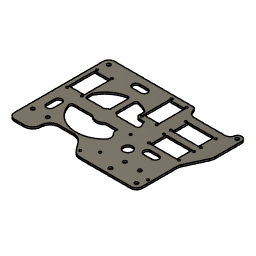
3_Superior (Autodesk Fusion 360 design; units mm, degrees)
Autodesk Fusion 360 part; units mm, degrees
sketch "Sketch1" plane through (0, 0, 0) normal (0, 1, 0) x (1, 0, 0)
  line L0 (40.357, -84) -> (129, -84)
  circle A0 centre (134, -59) radius 2
  arc A1 (35.9352, -34.7659) -> (35.1217, -20.107) centre (28.7481, -27.8127) ccw
  circle A2 centre (31, -74) radius 2
  arc A3 (129, -84) -> (139, -74) centre (129, -74) ccw
  circle A4 centre (51, -59) radius 2
  arc A5 (28.5369, -78.2349) -> (40.357, -84) centre (40.357, -69) ccw
  line L1 (11.1803, -10) -> (32.2785, -10)
  circle A6 centre (129, -74) radius 3
  arc A7 (32.2785, -10) -> (35.1217, -20.107) centre (41, -13) ccw
  circle A8 centre (-73, -52) radius 3
  arc A9 (-56, -84) -> (-41, -69) centre (-56, -69) ccw
  circle A10 centre (-73, 80) radius 3
  line L2 (-83, 80) -> (-83, -74)
  line L3 (-5, 45.111) -> (-5, 14.1421)
  arc A11 (9.7826, 49.0337) -> (5, 45.111) centre (9, 45.111) ccw
  arc A12 (-5, 14.1421) -> (-11.1803, 10) centre (0, 0) ccw
  arc A13 (-44.3962, 10.042) -> (-43.8178, 10) centre (-43.8178, 14) ccw
  arc A14 (-83, -74) -> (-73, -84) centre (-73, -74) ccw
  arc A15 (15.608, -61.6868) -> (-0.1522, -54) centre (-0.1522, -74) ccw
  arc A16 (-11.1803, -10) -> (11.1803, -10) centre (0, 0) ccw
  line L4 (63.3347, 90) -> (-73, 90)
  line L5 (-11.1803, 10) -> (-41.3962, 10)
  arc A17 (-5, 45.111) -> (-9.7826, 49.0337) centre (-9, 45.111) ccw
  line L6 (-73, -84) -> (-56, -84)
  line L7 (-68.3571, -32.6664) -> (-68.3571, -18.3202)
  circle A18 centre (-47, -52) radius 3
  arc A19 (-68.3571, -32.6664) -> (-56.1475, -32.6664) centre (-62.2523, -32.6664) ccw
  line L8 (-43.8178, -10) -> (-11.1803, -10)
  line L9 (43.8178, 10) -> (11.1803, 10)
  arc A20 (43.8178, 10) -> (47.628, 15.2174) centre (43.8178, 14) ccw
  circle A21 centre (51, -6) radius 2
  line L10 (15.608, -61.6868) -> (28.5369, -78.2349)
  circle A22 centre (84, -74) radius 3
  arc A23 (-26, -54) -> (-41, -69) centre (-26, -69) ccw
  line L11 (-56.1475, -18.3202) -> (-56.1475, -32.6664)
  arc A24 (-9.7826, 49.0337) -> (-44.3962, 22.9996) centre (0, 0) ccw
  arc A25 (-56.1475, -18.3202) -> (-68.3571, -18.3202) centre (-62.2523, -18.3202) ccw
  arc A26 (11.1803, 10) -> (5, 14.1421) centre (0, 0) ccw
  line L12 (5, 14.1421) -> (5, 45.111)
  arc A27 (-43.8178, -10) -> (-47.628, -15.2174) centre (-43.8178, -14) ccw
  line L13 (-26, -54) -> (-0.1522, -54)
  arc A28 (-47.628, -15.2174) -> (35.9352, -34.7659) centre (0, 0) ccw
  arc A29 (-73, 90) -> (-83, 80) centre (-73, 80) ccw
  circle A30 centre (150, 80) radius 3
  line L14 (67.95, 86.9234) -> (70.7446, 80.2178)
  arc A31 (70.7446, 80.2178) -> (80.7256, 74.43) centre (80.7256, 85.93) ccw
  line L15 (80.7256, 74.43) -> (134, 74.43)
  arc A32 (134, 74.43) -> (143.5, 83.93) centre (134, 83.93) ccw
  line L16 (157.5957, 80) -> (157.5957, 34.3748)
  line L17 (155.7692, 26.0247) -> (140.8265, -6.4974)
  line L18 (139, -74) -> (139, -14.8474)
  arc A33 (67.95, 86.9234) -> (63.3347, 90) centre (63.3347, 85) ccw
  arc A34 (155.7692, 26.0247) -> (157.5957, 34.3748) centre (137.5957, 34.3748) ccw
  arc A35 (140.8265, -6.4974) -> (139, -14.8474) centre (159, -14.8474) ccw
  arc A36 (157.5957, 80) -> (143.5, 83.93) centre (150, 80) ccw
  arc A37 (78.8091, 65.3966) -> (73.3091, 59.8966) centre (78.8091, 59.8966) ccw construction
  line L19 (73.3091, 59.8966) -> (73.3091, 36.8966) construction
  arc A38 (73.3091, 36.8966) -> (78.8091, 31.3966) centre (78.8091, 36.8966) ccw construction
  line L20 (78.8091, 31.3966) -> (131.8091, 31.3966) construction
  arc A39 (131.8091, 31.3966) -> (137.3091, 36.8966) centre (131.8091, 36.8966) ccw construction
  line L21 (137.3091, 36.8966) -> (137.3091, 59.8966) construction
  arc A40 (137.3091, 59.8966) -> (131.8091, 65.3966) centre (131.8091, 59.8966) ccw construction
  line L22 (131.8091, 65.3966) -> (78.8091, 65.3966) construction
  line L23 (127.8091, 61.8966) -> (82.8091, 61.8966)
  line L24 (82.8091, 61.8966) -> (82.8091, 34.8966)
  line L25 (82.8091, 34.8966) -> (127.8091, 34.8966)
  line L26 (127.8091, 34.8966) -> (127.8091, 61.8966)
  line L27 (73.3091, 21.8966) -> (73.3091, -1.1034) construction
  arc A41 (78.8091, 27.3966) -> (73.3091, 21.8966) centre (78.8091, 21.8966) ccw construction
  line L28 (131.8091, 27.3966) -> (78.8091, 27.3966) construction
  arc A42 (137.3091, 21.8966) -> (131.8091, 27.3966) centre (131.8091, 21.8966) ccw construction
  line L29 (137.3091, -1.1034) -> (137.3091, 21.8966) construction
  arc A43 (131.8091, -6.6034) -> (137.3091, -1.1034) centre (131.8091, -1.1034) ccw construction
  line L30 (78.8091, -6.6034) -> (131.8091, -6.6034) construction
  arc A44 (73.3091, -1.1034) -> (78.8091, -6.6034) centre (78.8091, -1.1034) ccw construction
  line L31 (127.8091, -3.1034) -> (127.8091, 23.8966)
  line L32 (127.8091, 23.8966) -> (82.8091, 23.8966)
  line L33 (82.8091, 23.8966) -> (82.8091, -3.1034)
  line L34 (82.8091, -3.1034) -> (127.8091, -3.1034)
  line L35 (34.3073, 25.1533) -> (57.3073, 25.1533) construction
  arc A45 (57.3073, 25.1533) -> (62.8073, 30.6533) centre (57.3073, 30.6533) ccw construction
  line L36 (62.8073, 30.6533) -> (62.8073, 83.6533) construction
  arc A46 (62.8073, 83.6533) -> (57.3073, 89.1533) centre (57.3073, 83.6533) ccw construction
  line L37 (57.3073, 89.1533) -> (34.3073, 89.1533) construction
  line L38 (28.8073, 83.6533) -> (28.8073, 30.6533) construction
  arc A47 (34.3073, 89.1533) -> (28.8073, 83.6533) centre (34.3073, 83.6533) ccw construction
  arc A48 (28.8073, 30.6533) -> (34.3073, 25.1533) centre (34.3073, 30.6533) ccw
  line L39 (59.4008, 79.7859) -> (32.4008, 79.7859)
  line L40 (32.4008, 79.7859) -> (32.4008, 34.7859)
  line L41 (32.4008, 34.7859) -> (59.4008, 34.7859)
  line L42 (59.4008, 34.7859) -> (59.4008, 79.7859)
  line L43 (28.8073, 30.6533) -> (28.8073, 40.8674)
  line L44 (34.3073, 25.1533) -> (43.2124, 25.1533)
  line L45 (-50.9384, 67.8681) -> (-73.9384, 67.8681) construction
  arc A49 (-73.9384, 67.8681) -> (-79.4384, 62.3681) centre (-73.9384, 62.3681) ccw construction
  line L46 (-79.4384, 62.3681) -> (-79.4384, 9.3681) construction
  arc A50 (-79.4384, 9.3681) -> (-73.9384, 3.8681) centre (-73.9384, 9.3681) ccw construction
  line L47 (-73.9384, 3.8681) -> (-50.9384, 3.8681) construction
  line L48 (-45.4384, 9.3681) -> (-45.4384, 62.3681) construction
  arc A51 (-50.9384, 3.8681) -> (-45.4384, 9.3681) centre (-50.9384, 9.3681) ccw construction
  arc A52 (-45.4384, 62.3681) -> (-50.9384, 67.8681) centre (-50.9384, 62.3681) ccw construction
  line L49 (-75.9384, 13.3681) -> (-48.9384, 13.3681)
  line L50 (-48.9384, 13.3681) -> (-48.9384, 58.3681)
  line L51 (-48.9384, 58.3681) -> (-75.9384, 58.3681)
  line L52 (-75.9384, 58.3681) -> (-75.9384, 13.3681)
  circle A53 centre (-86.6447, -5.091) radius 2
  line L53 (92.2002, -12.6067) -> (106.5464, -12.6067)
  arc A54 (106.5464, -24.8162) -> (106.5464, -12.6067) centre (106.5464, -18.7114) ccw
  line L54 (106.5464, -24.8162) -> (92.2002, -24.8162)
  arc A55 (92.2002, -12.6067) -> (92.2002, -24.8162) centre (92.2002, -18.7114) ccw
  circle A56 centre (87, -52) radius 3
  circle A57 centre (113, -52) radius 3
  circle A58 centre (70, -30) radius 8.1749
  line L55 (105.3091, 61.8966) -> (105.3091, 35) construction
  line L56 (105.3091, -3.1034) -> (105.3091, 23.8966) construction
  circle A59 centre (79.3091, 23.3966) radius 2
  circle A60 centre (79.3091, -2.6034) radius 2
  circle A61 centre (131.3091, -2.6034) radius 2
  circle A62 centre (131.3091, 23.3966) radius 2
  circle A63 centre (131.3091, 35.4483) radius 2
  circle A64 centre (79.3091, 61.4483) radius 2
  circle A65 centre (79.3091, 35.4483) radius 2
  circle A66 centre (131.3091, 61.4483) radius 2
  circle A67 centre (58.9008, 31.2859) radius 2
  circle A68 centre (58.9008, 83.2859) radius 2
  circle A69 centre (32.9008, 31.2859) radius 2
  circle A70 centre (32.9008, 83.2859) radius 2
  circle A71 centre (-75.4384, 61.8681) radius 2
  circle A72 centre (-75.4384, 9.8681) radius 2
  circle A73 centre (-49.4384, 9.8681) radius 2
  circle A74 centre (-49.4384, 61.8681) radius 2
  arc A75 (47.628, 15.2174) -> (43.2124, 25.1533) centre (0, 0) ccw
  arc A76 (28.8073, 40.8674) -> (9.7826, 49.0337) centre (0, 0) ccw
  line L57 (-44.3962, 13) -> (-44.3962, 22.9996)
  arc A77 (-44.3962, 13) -> (-41.3962, 10) centre (-41.3962, 13) ccw
  line L58 (-17.3077, 77.5267) -> (-2.9615, 77.5267)
  line L59 (-2.9615, 65.3172) -> (-17.3077, 65.3172)
  arc A78 (-17.3077, 77.5267) -> (-17.3077, 65.3172) centre (-17.3077, 71.422) ccw
  arc A79 (-2.9615, 65.3172) -> (-2.9615, 77.5267) centre (-2.9615, 71.422) ccw
  point P0 (32.9008, 29.2859)
  point P1 (-50.9614, 82.5095)
  point P2 (-60.6447, 50.909)
  point P3 (105.3091, 48.4483)
  point P4 (105.3091, 10.3966)
  point P5 (105.3091, 10.3966)
  point P6 (105.3091, 48.4483)
  point P7 (45.9008, 57.2859)
  dimension "d4" = 5
  dimension "d5" = 20
  dimension "d6" = 20
  dimension "d8" = 45
  dimension "d9" = 27
  dimension "d12" = 45
  dimension "d13" = 27
  dimension "d14" = 45
  dimension "d15" = 27
  dimension "d17" = 45
  dimension "d18" = 27
  dimension "d23" = 3
  constraint tangent A31 L15
  constraint tangent L15 A32
  constraint concentric A30 A36
  constraint tangent L16 A36
  constraint vertical L16
  constraint tangent L4 A33
  constraint tangent L14 A33
  constraint tangent L17 A34
  constraint tangent L16 A34
  constraint tangent L18 A35
  constraint tangent L17 A35
  constraint horizontal L23
  constraint perpendicular L23 L24
  constraint parallel L23 L25
  constraint parallel L24 L26
  constraint horizontal L32
  constraint perpendicular L32 L33
  constraint parallel L32 L34
  constraint parallel L31 L33
  constraint perpendicular L40 L41
  constraint parallel L40 L42
  constraint parallel L39 L41
  constraint coincident L43.end A75
  constraint coincident L38 L43.end
  constraint tangent A48 L43
  constraint coincident L35 L44.end
  constraint tangent A48 L44
  constraint perpendicular L50 L51
  constraint parallel L50 L52
  constraint parallel L49 L51
  constraint midpoint L23 L55.start
  constraint perpendicular L23 L55
  constraint midpoint L32 L56.end
  constraint midpoint L34 L56.start
  constraint midpoint L55 P6
  constraint midpoint L56 P5
  constraint concentric A75 A76
  constraint parallel L48 L57
  constraint coincident A13.end L5
  constraint coincident A13.start L57
  constraint tangent L5 A77
  constraint tangent L57 A77
  measures "d4" radius of A33
  measures "d5" radius of A34
  measures "d6" radius of A35
  measures "d8" distance of L25.end L24.end
  measures "d9" distance of L23.end L24.end
  measures "d12" distance of L31.start L33.end
  measures "d13" distance of L32.end L33.end
  measures "d14" distance of L39.start L41.end
  measures "d15" distance of L40.end L41.end
  measures "d17" distance of L49.start L51.end
  measures "d18" distance of L50.end L51.end
  measures "d23" radius of A77
extrude "Extrude1" add sketch "Sketch1" along normal blind 3 contours L0 A3 A5 A9 L2 A14 A15 L4 L6 L10 A23 L13 A29 L14 A31 L15 A32 L16 L17 L18 A33 A34 A35 A36
